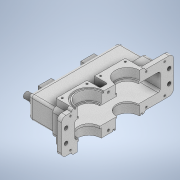
# Autodesk Inventor part: Gehäuse
Saved by Autodesk Inventor 2022 (Build 260153000, 153)
## iProperties
Created: 2023-01-26
Part Number: Gehäuse
Material: Aluminium 6061
Document SubType Name: Modeling
Designer: Matias Nicky
Density: 2.7 g/cm^3
Appearance: Aluminiumguss
Author: Matias Nicky
Autodesk Inventor part; units mm, degrees
ref_plane "XY Plane" through (0, 0, 0) normal (0, 0, 1) x (1, 0, 0)
sketch "Skizze1" plane through (0, 0, 0) normal (1, 0, 0) x (0, 1, 0)
  line L0 (-20, 102) -> (20, 102)
  line L1 (25, 97) -> (25, -97)
  line L2 (20, -102) -> (-20, -102)
  line L3 (-25, -97) -> (-25, 97)
  line L4 (-25, 102) -> (25, -102) construction
  line L5 (25, 102) -> (-25, -102) construction
  line L6 (-36.4497, 0) -> (36.4497, 0) projected
  arc A0 (25, 97) -> (20, 102) centre (20, 97) ccw
  arc A1 (-20, 102) -> (-25, 97) centre (-20, 97) ccw
  arc A2 (-25, -97) -> (-20, -102) centre (-20, -97) ccw
  arc A3 (20, -102) -> (25, -97) centre (20, -97) ccw
  point P0 (0, 0)
  dimension "d0" = 50
  dimension "d1" = 204
  dimension "d37" = 5
  dimension "d38" = 5
  constraints: 12 end point, 8 point on circle, 8 point on line, 8 tangent, 4 centre point, 2 equal radius, 2 midpoint, 2 parallel, 1 horizontal, 1 perpendicular, 1 other
  measures "d0" distance between parallel lines of L3 L1
  measures "d1" distance between parallel lines of L2 L0
  measures "d37" radius of A0
  measures "d38" radius of A1
extrude "Extrusion1" add sketch "Skizze1" along normal blind 102
sketch "Skizze2" plane through (102, 0, 0) normal (1, 0, 0) x (0, 0, -1)
  line L0 (-97, -20) -> (97, -20)
  line L1 (97, -20) -> (97, 20)
  line L2 (97, 20) -> (-97, 20)
  line L3 (-97, 20) -> (-97, -20)
  line L4 (-97, -20) -> (97, 20) construction
  line L5 (97, -20) -> (-97, 20) construction
  line L6 (177.8, 0) -> (-177.8, 0) projected
  point P0 (0, 0)
  dimension "d4" = 194
  dimension "d5" = 40
  constraints: 12 end point, 2 midpoint, 2 parallel, 1 horizontal, 1 perpendicular
  measures "d4" distance of L2.end L1.end
  measures "d5" distance between parallel lines of L0 L2
extrude "Extrusion2" cut sketch "Skizze2" against normal blind 97
ref_plane "Arbeitsebene1" through (102, 0, 0) normal (1, 0, 0) x (0, 1, 0)
fillet "Rundung3" radius 5 1 edges at (53.5, 20, 97)
fillet "Rundung4" radius 5 8 edges at (53.5, -20, 97) (53.5, -20, -97) (53.5, 20, -97) (5, 18.5355, 95.5355) (5, -2.5, 97) (5, 20, -2.5) (5, 0, -97) (5, -20, 0)
fillet "Rundung5" radius 10 8 edges at (0, 25, 0) (0, 23.5355, 100.5355) (0, 0, 102) (0, -23.5355, 100.5355) (0, -25, 0) (0, -23.5355, -100.5355) (0, 0, -102) (0, 23.5355, -100.5355)
sketch "Skizze5" plane through (102, 0, 0) normal (1, 0, 0) x (0, 1, 0)
  line L0 (-20, -102) -> (20, -102)
  line L1 (25, -97) -> (25, 97)
  line L2 (20, 102) -> (-20, 102)
  line L3 (-25, 97) -> (-25, -97)
  arc A0 (25, 97) -> (20, 102) centre (20, 97) ccw
  arc A1 (-20, 102) -> (-25, 97) centre (-20, 97) ccw
  arc A2 (-25, -97) -> (-20, -102) centre (-20, -97) ccw
  arc A3 (20, -102) -> (25, -97) centre (20, -97) ccw
  line L4 (40, 127) -> (40, 104.403)
  line L5 (40, 104.403) -> (45, 104.403)
  line L6 (45, -62.597) -> (40, -62.597)
  line L7 (-40, 127) -> (-40, 104.403)
  line L8 (-40, 104.403) -> (-45, 104.403)
  line L9 (-45, 104.403) -> (-45, 24.403)
  line L10 (-45, 17.403) -> (-45, -62.597)
  line L11 (-45, -62.597) -> (-40, -62.597)
  line L12 (-40, -62.597) -> (-40, -127)
  line L13 (25, 97) -> (25, -97) projected
  line L14 (-15, 97) -> (15, 97) projected
  line L15 (45, -62.597) -> (45, -22.597)
  line L16 (45, -22.597) -> (45, 17.403)
  line L17 (45, 24.403) -> (45, 64.403)
  line L18 (45, 64.403) -> (45, 104.403)
  line L19 (15, -97) -> (-15, -97) projected
  line L20 (40, -62.597) -> (40, -127)
  line L21 (40, 127) -> (-40, 127)
  line L22 (40, -127) -> (-40, -127)
  line L23 (-105, 0) -> (105, 0) projected
  line L24 (-45, 24.403) -> (-45, 17.403)
  line L25 (45, 24.403) -> (45, 17.403)
  line L26 (0, -177.8) -> (0, 177.8) projected
  point P0 (0, 0)
  dimension "d46" = 5
  dimension "d85" = 80
  dimension "d116" = 254
  dimension "d118" = 80
  dimension "d119" = 80
  dimension "d121" = 80
  dimension "d122" = 80
  dimension "d123" = 32.597
  dimension "d322" = 80
  dimension "d323" = 5
  constraints: 44 end point, 10 equal length, 8 point on circle, 8 tangent, 6 vertical, 5 perpendicular, 4 centre point, 3 equal radius, 2 point on line, 1 horizontal, 3 other
  measures "d46" radius of A0
  measures "d85" distance between parallel lines of L12 L20
  measures "d116" distance between parallel lines of L22 L21
  measures "d118" distance of L10.start L10.end
  measures "d119" distance of L8.end L9.end
  measures "d121" distance from line of L16.end L6
  measures "d122" distance of L5.end L17.start
  measures "d123" distance from line of L14 L17.end
  measures "d322" distance between parallel lines of L7 L4
  measures "d323" distance between parallel lines of L4 L18
extrude "Extrusion5" add sketch "Skizze5" against normal blind 40 contours L0 L26 L22 L12 L11 L10 L23 L3 A2 | L0 A3 L1 L23 L16 L15 L6 L20 L22 L26 | L23 L10 L24 L9 L8 L7 L21 L26 L2 A1 L3 | L1 A0 L2 L26 L21 L4 L5 L18 L17 L25 L16 L23
ref_plane "Arbeitsebene2" through (0, 50, 0) normal (0, 1, 0) x (-1, 0, 0)
sketch "Skizze13" plane through (0, 0, 0) normal (-1, 0, 0) x (0, 0, 1)
  line L0 (63.5, -12.5) -> (33.5, -12.5)
  line L1 (33.5, -12.5) -> (33.5, 12.5)
  line L2 (33.5, 12.5) -> (63.5, 12.5)
  line L3 (63.5, 12.5) -> (63.5, -12.5)
  line L4 (63.5, -12.5) -> (33.5, 12.5) construction
  line L5 (33.5, -12.5) -> (63.5, 12.5) construction
  line L6 (-33.5, -12.5) -> (-63.5, -12.5)
  line L7 (-63.5, -12.5) -> (-63.5, 12.5)
  line L8 (-63.5, 12.5) -> (-33.5, 12.5)
  line L9 (-33.5, 12.5) -> (-33.5, -12.5)
  line L10 (-33.5, -12.5) -> (-63.5, 12.5) construction
  line L11 (-63.5, -12.5) -> (-33.5, 12.5) construction
  point P0 (0, 0)
  point P1 (48.5, 0)
  point P2 (-48.5, 0)
  dimension "d95" = 30
  dimension "d96" = 25
  dimension "d97" = 30
  dimension "d98" = 25
  dimension "d99" = 48.5
  dimension "d100" = 48.5
  constraints: 24 end point, 4 midpoint, 4 parallel, 2 horizontal, 2 perpendicular
  measures "d95" distance of L1.end L2.end
  measures "d96" distance of L0.end L1.end
  measures "d97" distance of L7.end L8.end
  measures "d98" distance of L6.end L7.end
  measures "d99" distance of point (48.5, 0) point (0, 0)
  measures "d100" distance of point (-48.5, 0) point (0, 0)
extrude "Extrusion11" add sketch "Skizze13" along normal blind 15
fillet "Rundung11" radius 10 4 edges at (82, 40, 127) (82, -40, 127) (82, -40, -127) (82, 40, -127)
sketch "Skizze20" plane through (102, -45, -62.597) normal (0, -1, 0) x (1, 0, 0)
  line L0 (0, 154.597) -> (0, -29.403) projected
  circle A0 centre (0, 127) radius 24.5
  line L1 (0, 167) -> (0, 0) projected
  circle A1 centre (0, 40) radius 24.5
  point P0 (-102, 62.597)
  point P1 (0, 159.597)
  point P2 (0, 15.5)
  point P3 (0, 64.5)
  point P4 (0, 102.5)
  point P5 (0, 151.5)
  dimension "d134" = 32.597
  dimension "d135" = 49
  dimension "d136" = 87
  constraints: 2 centre point, 2 point on line, 1 equal radius
  measures "d134" distance of A0.centre point (0, 159.597)
  measures "d135" diameter of A1
  measures "d136" distance of A1.centre A0.centre
extrude "Extrusion18" cut sketch "Skizze20" against normal through all contours L0 A0 | L0 A1 picked at (-9.3243, 120.8872) picked at (-11.4312, 41.9605)
sketch "Skizze21" plane through (62, -45, 104.403) normal (0, -1, 0) x (1, 0, 0)
  arc A0 (40, -15.5) -> (40, -64.5) centre (40, -40) ccw projected
  circle A1 centre (40, -40) radius 27.5
  point P0 (-62, -104.403)
  dimension "d139" = 55
  constraints: 1 centre point, 1 coincident
  measures "d139" diameter of A1
extrude "Extrusion19" cut sketch "Skizze21" against normal blind 20
sketch "Skizze22" plane through (62, -45, 104.403) normal (0, -1, 0) x (1, 0, 0)
  arc A0 (40, -102.5) -> (40, -151.5) centre (40, -127) ccw projected
  circle A1 centre (40, -127) radius 27.5
  point P0 (-62, -104.403)
  dimension "d142" = 55
  constraints: 1 centre point, 1 coincident
  measures "d142" diameter of A1
extrude "Extrusion20" cut sketch "Skizze22" against normal blind 22
sketch "Skizze23" plane through (62, 45, -62.597) normal (0, 1, 0) x (1, 0, 0)
  arc A0 (40, -15.5) -> (40, -64.5) centre (40, -40) ccw projected
  circle A1 centre (40, -40) radius 27.5
  point P0 (-62, -62.597)
  dimension "d145" = 55
  constraints: 1 centre point, 1 coincident
  measures "d145" diameter of A1
extrude "Extrusion21" cut sketch "Skizze23" against normal blind 20
sketch "Skizze24" plane through (62, 45, -62.597) normal (0, 1, 0) x (1, 0, 0)
  arc A0 (40, -102.5) -> (40, -151.5) centre (40, -127) ccw projected
  circle A1 centre (40, -127) radius 27.5
  point P0 (-62, -62.597)
  dimension "d148" = 55
  constraints: 1 centre point, 1 coincident
  measures "d148" diameter of A1
extrude "Extrusion22" cut sketch "Skizze24" against normal blind 22
sketch "Skizze27" plane through (62, 45, -62.597) normal (0, 1, 0) x (1, 0, 0)
  circle A0 centre (40, -127) radius 30
  circle A1 centre (40, -127) radius 33.55
  point P0 (-62, -62.597)
  dimension "d244" = 60
  dimension "d245" = 67.1
  constraints: 2 centre point, 2 coincident
  measures "d244" diameter of A0
  measures "d245" diameter of A1
sketch "Skizze28" plane through (62, -45, 104.403) normal (0, -1, 0) x (1, 0, 0)
  arc A0 (40, -99.5) -> (40, -154.5) centre (40, -127) ccw projected
  circle A1 centre (40, -127) radius 30
  circle A2 centre (40, -127) radius 33.55
  point P0 (-62, -104.403)
  dimension "d165" = 60
  dimension "d166" = 67.1
  constraints: 2 centre point, 2 coincident
  measures "d165" diameter of A1
  measures "d166" diameter of A2
extrude "Extrusion27" cut sketch "Skizze28" against normal blind 3.55
sketch "Skizze29" plane through (62, 0, 0) normal (-1, 0, 0) x (0, 0, 1)
  line L0 (127, -30) -> (127, 30) projected
  line L1 (127, 0) -> (127, -30)
  line L2 (127, -30) -> (127, -40)
  arc A0 (117, -40) -> (127, -30) centre (117, -30) ccw projected
  line L3 (127, -40) -> (117, -40)
  line L4 (104.403, -40) -> (117, -40) projected
  line L5 (104.403, -45) -> (104.403, -40) projected
  line L6 (104.403, -40) -> (104.403, -45)
  line L7 (104.403, -45) -> (99.403, -45)
  line L8 (99.403, -45) -> (99.403, -30)
  line L9 (99.403, -30) -> (107, -30)
  line L10 (127, 0) -> (127, 30)
  line L11 (127, 40) -> (127, 30)
  line L12 (104.403, 40) -> (104.403, 45) projected
  line L13 (104.403, 40.4013) -> (104.403, 45)
  line L14 (104.403, 45) -> (99.403, 45)
  line L15 (99.403, 45) -> (99.403, 30)
  line L16 (99.403, 30) -> (107, 30)
  line L17 (107, 30) -> (107, -30)
  line L18 (-62.597, 45) -> (-57.597, 45)
  line L19 (-62.597, 45) -> (-62.597, 40) projected
  line L20 (-62.597, 45) -> (-62.597, 40)
  line L21 (-62.597, 40) -> (-117, 40) projected
  line L22 (-62.597, 40) -> (-117, 40)
  line L23 (-117, 40) -> (-127, 40)
  line L24 (-127, 40) -> (-127, 30)
  line L25 (-127, 30) -> (-127, -30) projected
  line L26 (-127, 30) -> (-127, -30)
  line L27 (-127, -30) -> (-127, -40)
  line L28 (-127, -40) -> (-117, -40)
  line L29 (-117, -40) -> (-62.597, -40) projected
  line L30 (-117, -40) -> (-62.597, -40)
  line L31 (-62.597, -40) -> (-62.597, -45) projected
  line L32 (-62.597, -40) -> (-62.597, -45)
  line L33 (-62.597, -45) -> (104.403, -45) projected
  line L34 (-57.597, -30) -> (-57.597, -45)
  line L35 (-57.597, -30) -> (-107, -30)
  line L36 (-107, -30) -> (-107, 30)
  line L37 (-107, 30) -> (-57.597, 30)
  line L38 (-57.597, 45) -> (-57.597, 30)
  line L39 (29.403, -45) -> (12.403, -45)
  line L40 (12.403, -45) -> (12.403, -30)
  line L41 (29.403, -30) -> (29.403, -45)
  line L42 (104.403, 45) -> (-62.597, 45) projected
  line L43 (29.403, 45) -> (12.403, 45)
  line L44 (12.403, 45) -> (12.403, 30)
  line L45 (12.403, 30) -> (29.403, 30)
  line L46 (29.403, 30) -> (29.403, 45)
  line L47 (117, 40) -> (104.403, 40) projected
  line L48 (104.403, 40) -> (117, 40)
  line L49 (117, 40) -> (127, 40)
  line L50 (-62.597, -45) -> (-57.597, -45)
  line L51 (12.403, -30) -> (29.403, -30)
  point P0 (0, 0)
  point P1 (12.403, -45)
  point P2 (104.403, 40.4013)
  point P3 (12.403, 45)
  point P4 (104.403, 40.4095)
  dimension "d169" = 5
  dimension "d170" = 5
  dimension "d171" = 5
  dimension "d172" = 15
  dimension "d173" = 15
  dimension "d175" = 20
  dimension "d176" = 15
  dimension "d177" = 20
  dimension "d178" = 5
  dimension "d180" = 15
  dimension "d181" = 70
  dimension "d182" = 70
  dimension "d185" = 17
  dimension "d186" = 15
  dimension "d187" = 70
  constraints: 80 end point, 11 collinear, 10 perpendicular, 7 point on line, 5 horizontal, 4 parallel, 2 vertical, 1 midpoint, 1 point on circle, 1 tangent
  measures "d169" distance of L5.start L7.end
  measures "d170" distance of L12.end L14.end
  measures "d171" distance of L18.start L18.end
  measures "d172" distance of L14.end L15.end
  measures "d173" distance of L7.end L8.end
  measures "d175" distance between parallel lines of L0 L17
  measures "d176" distance between parallel lines of L18 L37
  measures "d177" distance between parallel lines of L25 L36
  measures "d178" distance from line of L31.end L34
  measures "d180" distance between parallel lines of L35 L33
  measures "d181" distance between parallel lines of L8 L41
  measures "d182" distance between parallel lines of L40 L34
  measures "d185" distance of L44.end L45.end
  measures "d186" distance of L45.end L43.start
  measures "d187" distance between parallel lines of L38 L44
extrude "Extrusion28" cut sketch "Skizze29" against normal blind 30 contours A0 L4 L5 L7 L8 L9 L17 L16 L15 L14 L12 L47 L49 L11 L0 | L33 L40 L51 L41 | L33 L31 L29 L28 L27 L25 L24 L23 L21 L19 L18 L38 L37 L36 L35 L34 | L46 L45 L44 L42
sketch "Skizze30" plane through (92, 0, 0) normal (-1, 0, 0) x (0, 0, 1)
  arc A0 (117, -40) -> (127, -30) centre (117, -30) ccw projected
  line L0 (127, 30) -> (127, -30) projected
  line L1 (-178.2142, 0) -> (180.2853, 0) projected
  line L2 (29.403, -30) -> (29.403, -45) projected
  line L3 (29.403, -45) -> (12.403, -45) projected
  line L4 (12.403, 45) -> (29.403, 45) projected
  line L5 (12.403, 30) -> (12.403, 45) projected
  line L6 (-127, -30) -> (-127, 30) projected
  point P0 (0, 0)
  point P1 (117, -15)
  point P2 (117, 15)
  point P3 (-117, -15)
  point P4 (-117, 15)
  dimension "d188" = 30
  dimension "d189" = 10
  dimension "d190" = 10
  dimension "d191" = 15
  dimension "d196" = 10
  dimension "d197" = 10
  measures "d188" distance of point (117, 15) point (117, -15)
  measures "d189" distance from line of L0 point (117, -15)
  measures "d190" distance from line of L0 point (117, 15)
  measures "d191" distance from line of point (117, 15) L1
  measures "d196" distance from line of L6 point (-117, -15)
  measures "d197" distance from line of L6 point (-117, 15)
fillet "Rundung12" radius 10 4 edges at (77, 30, 107) (77, -30, 107) (77, 30, -107) (77, -30, -107)
hole "Bohrung1" at (92, -15, 117) at (92, 15, 117) at (92, -15, -117) at (92, 15, -117) direction (1, 0, 0) diameter 8.376 depth 27.3 thread size "M10x1.5" class "6H" standard "ANSI Metric M Profile"
sketch "Skizze31" plane through (102, 0, 0) normal (1, 0, 0) x (0, 0, -1)
  line L0 (-91.903, 23) -> (-91.903, 45) projected
  line L1 (-104.403, 40) -> (-117, 40) projected
  line L2 (50.097, 45) -> (50.097, 25) projected
  line L3 (117, 40) -> (62.597, 40) projected
  line L4 (50.097, -23) -> (50.097, -45) projected
  line L5 (62.597, -40) -> (117, -40) projected
  line L6 (-97, -15) -> (-97, 15) projected
  line L7 (-91.903, -45) -> (-91.903, -25) projected
  line L8 (-117, -40) -> (-104.403, -40) projected
  line L9 (97, 15) -> (97, -15) projected
  point P0 (0, 0)
  point P1 (-107, 33.5)
  point P2 (65.097, 35)
  point P3 (65.097, -35)
  point P4 (-91.903, 20)
  point P5 (50.097, -20)
  point P6 (-107, -33.5)
  point P7 (107, 33.5)
  point P8 (107, -33.5)
  dimension "d207" = 6.5
  dimension "d208" = 15
  dimension "d211" = 15
  dimension "d212" = 5
  dimension "d235" = 10
  dimension "d237" = 10
  dimension "d238" = 6.5
  dimension "d239" = 10
  dimension "d240" = 6.5
  dimension "d241" = 6.5
  dimension "d324" = 5
  measures "d207" distance from line of L1 point (-107, 33.5)
  measures "d208" distance from line of point (65.097, 35) L2
  measures "d211" distance from line of L4 point (65.097, -35)
  measures "d212" distance from line of L5 point (65.097, -35)
  measures "d235" distance from line of point (-107, 33.5) L6
  measures "d237" distance from line of point (-107, -33.5) L6
  measures "d238" distance from line of L8 point (-107, -33.5)
  measures "d239" distance from line of point (107, 33.5) L9
  measures "d240" distance from line of L3 point (107, 33.5)
  measures "d241" distance from line of L5 point (107, -33.5)
  measures "d324" distance from line of L3 point (65.097, 35)
hole "Bohrung2" at (102, 33.5, 107) at (102, 35, -65.097) at (102, -35, -65.097) at (102, -33.5, 107) at (102, 33.5, -107) at (102, -33.5, -107) direction (-1, 0, 0) diameter 4.134 depth 14.2 thread size "M5x0.8" class "6H" standard "ANSI Metric M Profile"
fillet "Rundung14" radius 3 4 edges at (92, -37.5, 12.403) (92, -37.5, 29.403) (92, 37.5, 12.403) (92, 37.5, 29.403)
sketch "Skizze32" plane through (102, 0, 0) normal (1, 0, 0) x (0, 0, -1)
  line L0 (-4.903, 45) -> (50.097, 45) projected
  line L1 (-36.903, -45) -> (-10.953, -45) projected
  point P0 (0, 0)
  point P1 (-20.903, 37.5)
  point P2 (-30.853, 45.4092)
  point P3 (-12.403, 45)
  point P4 (-20.903, -37.5)
  point P5 (-12.403, -45)
  point P6 (50.097, 45)
  dimension "d224" = 7.5
  dimension "d226" = 7.5
  dimension "d242" = 8.5
  dimension "d243" = 8.5
  constraints: 1 other
  measures "d226" distance from line of point (-20.903, -37.5) L1
  measures "d242" horizontal distance of point (-12.403, -45) point (-20.903, -37.5)
  measures "d243" horizontal distance of point (-12.403, 45) point (-20.903, 37.5)
hole "Bohrung3" at (102, 37.5, 20.903) at (102, -37.5, 20.903) direction (-1, 0, 0) diameter 4.917 depth 17.1 thread size "M6x1" class "6H" standard "ANSI Metric M Profile"
extrude "Extrusion29" cut sketch "Skizze27" against normal blind 3.55
sketch "Skizze33" plane through (102, -45, 91.903) normal (0, -1, 0) x (1, 0, 0)
  line L0 (-40, -149.5) -> (-40, -79.5) projected
  line L1 (-13, -79.5) -> (-40, -79.5) projected
  line L2 (-40, -149.5) -> (-10, -149.5) projected
  line L3 (-40, -62.5) -> (-13, -62.5) projected
  line L4 (-40, -62.5) -> (-40, 7.5) projected
  line L5 (-10, 7.5) -> (-40, 7.5) projected
  point P0 (-102, -91.903)
  point P1 (-33, 0.5)
  point P2 (-33, -55.5)
  point P3 (-33, -86.5)
  point P4 (-33, -142.5)
  point P5 (-40, -154.5)
  point P6 (-40, 12.5)
  dimension "d248" = 7
  dimension "d249" = 7
  dimension "d250" = 7
  dimension "d251" = 7
  dimension "d252" = 7
  dimension "d253" = 7
  dimension "d254" = 7
  dimension "d255" = 7
  measures "d248" distance from line of L0 point (-33, -86.5)
  measures "d249" distance from line of L1 point (-33, -86.5)
  measures "d250" distance from line of L0 point (-33, -142.5)
  measures "d251" distance from line of L2 point (-33, -142.5)
  measures "d252" distance from line of L3 point (-33, -55.5)
  measures "d253" distance from line of L4 point (-33, -55.5)
  measures "d254" distance from line of L4 point (-33, 0.5)
  measures "d255" distance from line of L5 point (-33, 0.5)
hole "Bohrung4" at (69, -45, 92.403) at (69, -45, 36.403) at (69, -45, 5.403) at (69, -45, -50.597) direction (0, 1, 0) diameter 4.134 depth 14.2 thread size "M5x0.8" class "6H" standard "ANSI Metric M Profile"
sketch "Skizze34" plane through (102, 45, -50.097) normal (0, 1, 0) x (1, 0, 0)
  circle A0 centre (-33, -55.5) radius 2.067 projected
  circle A1 centre (-33, -86.5) radius 2.067 projected
  circle A2 centre (-33, -142.5) radius 2.067 projected
  circle A3 centre (-33, 0.5) radius 2.067 projected
  point P0 (-102, -50.097)
  point P1 (-33, -55.5)
  point P2 (-33, -86.5)
  point P3 (-33, -142.5)
  point P4 (-33, 0.5)
  constraints: 4 coincident
hole "Bohrung5" at (69, 45, 5.403) at (69, 45, 36.403) at (69, 45, 92.403) at (69, 45, -50.597) direction (0, -1, 0) diameter 4.134 depth 14.2 thread size "M5x0.8" class "6H" standard "ANSI Metric M Profile"
fillet "Rundung15" radius 5 4 edges at (97, 45, -62.597) (97, 45, 104.403) (97, -45, -62.597) (97, -45, 104.403)
sketch "Skizze35" plane through (0, 0, 0) normal (-1, 0, 0) x (0, 0, 1)
  circle A0 centre (82, 0) radius 10
  line L0 (-92, -15) -> (-92, 15) projected
  line L1 (92, 15) -> (92, -15) projected
  point P0 (0, 0)
  dimension "d271" = 20
  dimension "d289" = 10
  constraints: 1 centre point
  measures "d271" diameter of A0
  measures "d289" distance from line of L1 A0.centre
extrude "Extrusion30" add sketch "Skizze35" along normal blind 5
sketch "Skizze36" plane through (-5, 0, 82) normal (-1, 0, 0) x (0, 0, 1)
  circle A0 centre (0, 0) radius 10 projected
  circle A1 centre (0, 0) radius 7
  point P0 (-82, 0)
  point P1 (-10, 0)
  dimension "d275" = 14
  constraints: 1 centre point, 1 coincident, 1 horizontal alignment
  measures "d275" diameter of A1
extrude "Extrusion31" add sketch "Skizze36" along normal blind 18 contours A1
thread "Gewinde2" size "M14x2" class "6g" standard "ANSI Metric M Profile" length 29.966
sketch "Skizze37" plane through (-23, 0, 82) normal (-1, 0, 0) x (0, 0, 1)
  point P0 (-82, 0)
  point P1 (0, 0)
hole "Bohrung6" at (-23, 0, 82) direction (1, 0, 0) diameter 10 end through all
sketch "Skizze39" plane through (-15, 0, 0) normal (-1, 0, 0) x (0, 0, 1)
  line L0 (63.5, -12.5) -> (63.5, 12.5) projected
  line L1 (33.5, 12.5) -> (33.5, -12.5) projected
  line L2 (33.5, -12.5) -> (63.5, -12.5) projected
  line L3 (63.5, 12.5) -> (33.5, 12.5) projected
  line L4 (-33.5, -12.5) -> (-33.5, 12.5) projected
  line L5 (-63.5, -12.5) -> (-33.5, -12.5) projected
  line L6 (-63.5, 12.5) -> (-63.5, -12.5) projected
  line L7 (-33.5, 12.5) -> (-63.5, 12.5) projected
  point P0 (0, 0)
  point P1 (56, -6.25)
  point P2 (41, -6.25)
  point P3 (56, 6.25)
  point P4 (41, 6.25)
  point P5 (-41, -6.25)
  point P6 (-56, -6.25)
  point P7 (-56, 6.25)
  point P8 (-41, 6.25)
  dimension "d299" = 7.5
  dimension "d300" = 7.5
  dimension "d301" = 6.25
  dimension "d302" = 6.25
  dimension "d303" = 6.25
  dimension "d304" = 6.25
  dimension "d305" = 7.5
  dimension "d306" = 7.5
  dimension "d307" = 7.5
  dimension "d308" = 6.25
  dimension "d309" = 6.25
  dimension "d310" = 7.5
  dimension "d311" = 7.5
  dimension "d312" = 6.25
  dimension "d313" = 6.25
  dimension "d314" = 7.5
  measures "d299" distance from line of point (56, -6.25) L0
  measures "d300" distance from line of L1 point (41, -6.25)
  measures "d301" distance from line of L2 point (41, -6.25)
  measures "d302" distance from line of L2 point (56, -6.25)
  measures "d303" distance from line of L3 point (41, 6.25)
  measures "d304" distance from line of L3 point (56, 6.25)
  measures "d305" distance from line of point (41, 6.25) L1
  measures "d306" distance from line of L0 point (56, 6.25)
  measures "d307" distance from line of L4 point (-41, -6.25)
  measures "d308" distance from line of L5 point (-41, -6.25)
  measures "d309" distance from line of L5 point (-56, -6.25)
  measures "d310" distance from line of L6 point (-56, -6.25)
  measures "d311" distance from line of L6 point (-56, 6.25)
  measures "d312" distance from line of L7 point (-56, 6.25)
  measures "d313" distance from line of L7 point (-41, 6.25)
  measures "d314" distance from line of L4 point (-41, 6.25)
hole "Bohrung8" at (-15, -6.25, 56) at (-15, -6.25, 41) at (-15, 6.25, 56) at (-15, 6.25, 41) at (-15, -6.25, -41) at (-15, -6.25, -56) at (-15, 6.25, -56) at (-15, 6.25, -41) direction (1, 0, 0) diameter 4.134 depth 14.2 thread size "M5x0.8" class "6H" standard "ANSI Metric M Profile"
